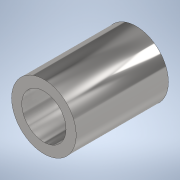
# Autodesk Inventor part: Для регулировки 1
Saved by Autodesk Inventor 2021 (Build 250183000, 183)
## iProperties
Created: 2020-12-19
Part Number: Для регулировки 1
Material: Сталь, высокопрочная, низколегированная
Document SubType Name: Modeling
Designer: Тимоха
Mass: 200.066 g
Surface Area: 102.871 cm^2
Volume: 25.4862 cm^3
Density: 7.85 g/cm^3
Appearance: Сталь — полированная
Author: Тимоха
Autodesk Inventor part; units mm, degrees
ref_plane "YZ Plane" through (0, 0, 0) normal (1, 0, 0) x (0, 1, 0)
ref_plane "XZ Plane" through (0, 0, 0) normal (0, 1, 0) x (-1, 0, 0)
ref_plane "XY Plane" through (0, 0, 0) normal (0, 0, 1) x (1, 0, 0)
sketch "Эскиз1" plane through (0, 0, 0) normal (0, 0, 1) x (1, 0, 0)
  circle A0 centre (0, 0) radius 12
  circle A1 centre (0, 0) radius 17.5
  dimension "d0" = 24
  dimension "d1" = 35
  constraints: 2 centre point, 2 coincident
  measures "d0" diameter of A0
  measures "d1" diameter of A1
extrude "Выдавливание1" add sketch "Эскиз1" along normal blind 50
